Autodesk Fusion 360 part; units mm, degrees
note: some values were not read from the file. Set by a fixed rule: which sketch regions a step uses.
(part 2 of 2)
sketch "Sketch14" plane through (0, 0, 1.5) normal (0, 0, 1) x (-1, 0, 0)
  line L0 (-6.1342, -0.2087) -> (-6.1342, -10.2087)
  line L1 (-6.1342, -10.2087) -> (-9.8859, -10.2087)
  spline S0 degree 3 poles (-9.8859, -10.2087) (-10.2332, -10.2024) (-10.8611, -10.1909) (-11.4553, -9.9911) (-11.7208, -9.9018) knots 0 0 0 0 0.103457 0.187012 0.187012 0.187012 0.187012
  spline S1 degree 3 poles (-11.7208, -9.9018) (-11.9396, -9.7883) (-12.3751, -9.5625) (-12.6625, -9.165) (-12.8054, -8.9673) knots 0 0 0 0 0.07283 0.144951 0.144951 0.144951 0.144951
  spline S2 degree 3 poles (-12.8054, -8.9673) (-12.9208, -8.7579) (-13.1471, -8.3471) (-13.1833, -7.8798) (-13.201, -7.6508) knots 0 0 0 0 0.070808 0.13889 0.13889 0.13889 0.13889
  spline S3 degree 3 poles (-13.201, -7.6508) (-13.186, -7.4393) (-13.1557, -7.0123) (-12.9546, -6.6342) (-12.8532, -6.4434) knots 0 0 0 0 0.062849 0.126897 0.126897 0.126897 0.126897
  spline S4 degree 3 poles (-12.8532, -6.4434) (-12.7177, -6.2615) (-12.4343, -5.881) (-12.0193, -5.6499) (-11.8027, -5.5293) knots 0 0 0 0 0.067255 0.140662 0.140662 0.140662 0.140662
  spline S5 degree 3 poles (-11.8027, -5.5293) (-12.0835, -5.4301) (-12.6217, -5.2399) (-13.009, -4.8219) (-13.1942, -4.6221) knots 0 0 0 0 0.087856 0.168343 0.168343 0.168343 0.168343
  spline S6 degree 3 poles (-13.1942, -4.6221) (-13.3375, -4.3958) (-13.6301, -3.9333) (-13.6667, -3.3868) (-13.6854, -3.1078) knots 0 0 0 0 0.079028 0.161462 0.161462 0.161462 0.161462
  spline S7 degree 3 poles (-13.6854, -3.1078) (-13.6733, -2.8786) (-13.6495, -2.4244) (-13.4728, -2.0055) (-13.3852, -1.7981) knots 0 0 0 0 0.068285 0.135277 0.135277 0.135277 0.135277
  spline S8 degree 3 poles (-13.3852, -1.7981) (-13.2857, -1.6126) (-13.0966, -1.2602) (-12.7972, -0.9957) (-12.6553, -0.8704) knots 0 0 0 0 0.062563 0.118877 0.118877 0.118877 0.118877
  spline S9 degree 3 poles (-12.6553, -0.8704) (-12.4947, -0.7664) (-12.1539, -0.5456) (-11.7635, -0.4324) (-11.5571, -0.3725) knots 0 0 0 0 0.057092 0.121161 0.121161 0.121161 0.121161
  spline S10 degree 3 poles (-11.5571, -0.3725) (-11.3145, -0.3248) (-10.7833, -0.2204) (-10.2416, -0.2129) (-9.9473, -0.2087) knots 0 0 0 0 0.074013 0.162103 0.162103 0.162103 0.162103
  line L2 (-9.9473, -0.2087) -> (-6.1342, -0.2087)
  line L3 (-22.6281, -2.3711) -> (-23.8423, -2.5621)
  spline S11 degree 3 poles (-23.8423, -2.5621) (-23.8868, -2.337) (-23.9714, -1.9101) (-24.2681, -1.5932) (-24.4084, -1.4434) knots 0 0 0 0 0.06728 0.127631 0.127631 0.127631 0.127631
  spline S12 degree 3 poles (-24.4084, -1.4434) (-24.591, -1.3302) (-24.9905, -1.0825) (-25.4621, -1.0644) (-25.7181, -1.0546) knots 0 0 0 0 0.063382 0.138705 0.138705 0.138705 0.138705
  spline S13 degree 3 poles (-25.7181, -1.0546) (-25.9704, -1.0603) (-26.4193, -1.0704) (-26.8045, -1.2966) (-26.9732, -1.3957) knots 0 0 0 0 0.074162 0.131971 0.131971 0.131971 0.131971
  spline S14 degree 3 poles (-26.9732, -1.3957) (-27.0925, -1.5129) (-27.3215, -1.738) (-27.3627, -2.0554) (-27.3825, -2.2074) knots 0 0 0 0 0.048606 0.09328 0.09328 0.09328 0.09328
  spline S15 degree 3 poles (-27.3825, -2.2074) (-27.3667, -2.3392) (-27.3348, -2.606) (-27.1264, -2.7761) (-27.021, -2.8622) knots 0 0 0 0 0.038259 0.077458 0.077458 0.077458 0.077458
  spline S16 degree 3 poles (-27.021, -2.8622) (-26.8755, -2.9276) (-26.472, -3.1087) (-26.0413, -3.2122) (-25.7659, -3.2783) knots 0 0 0 0 0.047763 0.132466 0.132466 0.132466 0.132466
  spline S17 degree 3 poles (-25.7659, -3.2783) (-25.3814, -3.3747) (-24.7446, -3.5343) (-24.1326, -3.7711) (-23.89, -3.865) knots 0 0 0 0 0.118742 0.196704 0.196704 0.196704 0.196704
  spline S18 degree 3 poles (-23.89, -3.865) (-23.7289, -3.9545) (-23.4161, -4.1282) (-23.2024, -4.4149) (-23.0987, -4.5539) knots 0 0 0 0 0.054583 0.105986 0.105986 0.105986 0.105986
  spline S19 degree 3 poles (-23.0987, -4.5539) (-23.0211, -4.7061) (-22.8648, -5.0127) (-22.8434, -5.3563) (-22.8327, -5.5293) knots 0 0 0 0 0.050651 0.102072 0.102072 0.102072 0.102072
  spline S20 degree 3 poles (-22.8327, -5.5293) (-22.8414, -5.6869) (-22.8585, -5.9984) (-22.9873, -6.2825) (-23.051, -6.4229) knots 0 0 0 0 0.046874 0.092701 0.092701 0.092701 0.092701
  spline S21 degree 3 poles (-23.051, -6.4229) (-23.1324, -6.5556) (-23.295, -6.8203) (-23.5372, -7.0148) (-23.6581, -7.1119) knots 0 0 0 0 0.046313 0.092439 0.092439 0.092439 0.092439
  spline S22 degree 3 poles (-23.6581, -7.1119) (-23.7685, -7.1813) (-24.0116, -7.3342) (-24.2859, -7.4198) (-24.4357, -7.4666) knots 0 0 0 0 0.038962 0.085789 0.085789 0.085789 0.085789
  spline S23 degree 3 poles (-24.4357, -7.4666) (-24.6065, -7.5104) (-24.9556, -7.5998) (-25.3158, -7.611) (-25.4998, -7.6167) knots 0 0 0 0 0.052716 0.107755 0.107755 0.107755 0.107755
  spline S24 degree 3 poles (-25.4998, -7.6167) (-25.7686, -7.6089) (-26.2779, -7.5942) (-26.7641, -7.4427) (-26.9937, -7.3711) knots 0 0 0 0 0.080215 0.152023 0.152023 0.152023 0.152023
  spline S25 degree 3 poles (-26.9937, -7.3711) (-27.1909, -7.2879) (-27.5579, -7.133) (-27.825, -6.8387) (-27.9487, -6.7026) knots 0 0 0 0 0.063304 0.117817 0.117817 0.117817 0.117817
  spline S26 degree 3 poles (-27.9487, -6.7026) (-28.0443, -6.5436) (-28.2527, -6.197) (-28.3298, -5.7992) (-28.3716, -5.5839) knots 0 0 0 0 0.055232 0.120418 0.120418 0.120418 0.120418
  line L4 (-28.3716, -5.5839) -> (-27.171, -5.4202)
  spline S27 degree 3 poles (-27.171, -5.4202) (-27.1329, -5.5947) (-27.0588, -5.9329) (-26.8127, -6.1757) (-26.6935, -6.2933) knots 0 0 0 0 0.052312 0.101441 0.101441 0.101441 0.101441
  spline S28 degree 3 poles (-26.6935, -6.2933) (-26.5405, -6.3846) (-26.2017, -6.5868) (-25.8057, -6.5999) (-25.5885, -6.6071) knots 0 0 0 0 0.052622 0.116544 0.116544 0.116544 0.116544
  spline S29 degree 3 poles (-25.5885, -6.6071) (-25.3414, -6.6051) (-24.9157, -6.6017) (-24.5391, -6.4085) (-24.3811, -6.3274) knots 0 0 0 0 0.072813 0.125434 0.125434 0.125434 0.125434
  spline S30 degree 3 poles (-24.3811, -6.3274) (-24.2758, -6.2342) (-24.0766, -6.058) (-24.0379, -5.796) (-24.0196, -5.6726) knots 0 0 0 0 0.040701 0.076975 0.076975 0.076975 0.076975
  spline S31 degree 3 poles (-24.0196, -5.6726) (-24.026, -5.5949) (-24.0388, -5.4386) (-24.1259, -5.3083) (-24.1697, -5.2429) knots 0 0 0 0 0.022989 0.046194 0.046194 0.046194 0.046194
  spline S32 degree 3 poles (-24.1697, -5.2429) (-24.2308, -5.1782) (-24.3646, -5.0367) (-24.5433, -4.9581) (-24.6403, -4.9154) knots 0 0 0 0 0.026422 0.05785 0.05785 0.05785 0.05785
  spline S33 degree 3 poles (-24.6403, -4.9154) (-24.7612, -4.8773) (-25.1203, -4.7642) (-25.4838, -4.6665) (-25.7249, -4.6017) knots 0 0 0 0 0.038027 0.112916 0.112916 0.112916 0.112916
  spline S34 degree 3 poles (-25.7249, -4.6017) (-26.0956, -4.5032) (-26.7095, -4.3403) (-27.3039, -4.1171) (-27.5394, -4.0287) knots 0 0 0 0 0.114967 0.190379 0.190379 0.190379 0.190379
  spline S35 degree 3 poles (-27.5394, -4.0287) (-27.7016, -3.9491) (-28.0185, -3.7937) (-28.242, -3.5207) (-28.3511, -3.3875) knots 0 0 0 0 0.053495 0.104527 0.104527 0.104527 0.104527
  spline S36 degree 3 poles (-28.3511, -3.3875) (-28.4366, -3.2329) (-28.6171, -2.9066) (-28.635, -2.5334) (-28.6444, -2.337) knots 0 0 0 0 0.052263 0.110368 0.110368 0.110368 0.110368
  spline S37 degree 3 poles (-28.6444, -2.337) (-28.6284, -2.1337) (-28.5957, -1.72) (-28.3883, -1.3603) (-28.2829, -1.1774) knots 0 0 0 0 0.060367 0.122834 0.122834 0.122834 0.122834
  spline S38 degree 3 poles (-28.2829, -1.1774) (-28.1475, -1.006) (-27.8666, -0.6506) (-27.4623, -0.4449) (-27.2529, -0.3384) knots 0 0 0 0 0.064709 0.134257 0.134257 0.134257 0.134257
  spline S39 degree 3 poles (-27.2529, -0.3384) (-27.0154, -0.2528) (-26.5218, -0.0751) (-25.9971, -0.0553) (-25.7249, -0.045) knots 0 0 0 0 0.075252 0.156416 0.156416 0.156416 0.156416
  spline S40 degree 3 poles (-25.7249, -0.045) (-25.2992, -0.0571) (-24.5301, -0.079) (-23.866, -0.4611) (-23.5694, -0.6317) knots 0 0 0 0 0.125349 0.226485 0.226485 0.226485 0.226485
  spline S41 degree 3 poles (-23.5694, -0.6317) (-23.3443, -0.8611) (-22.8656, -1.3493) (-22.7103, -2.0172) (-22.6281, -2.3711) knots 0 0 0 0 0.094587 0.201201 0.201201 0.201201 0.201201
  line L5 (-51.0387, -0.2087) -> (-51.0387, -10.2087)
  line L6 (-51.0387, -10.2087) -> (-52.2665, -10.2087)
  line L7 (-52.2665, -10.2087) -> (-52.2665, -0.2087)
  line L8 (-52.2665, -0.2087) -> (-51.0387, -0.2087)
  line L9 (-33.2147, -0.2087) -> (-33.2147, -7.4529)
  line L10 (-33.2147, -7.4529) -> (-34.4425, -7.4529)
  line L11 (-34.4425, -7.4529) -> (-34.4425, -0.2087)
  line L12 (-34.4425, -0.2087) -> (-33.2147, -0.2087)
  spline S42 degree 3 poles (-20.0769, -1.1023) (-19.8601, -0.9267) (-19.4552, -0.5985) (-18.9808, -0.3836) (-18.7604, -0.2838) knots 0 0 0 0 0.08329 0.155589 0.155589 0.155589 0.155589
  spline S43 degree 3 poles (-18.7604, -0.2838) (-18.545, -0.2142) (-18.106, -0.0722) (-17.6448, -0.0542) (-17.4098, -0.045) knots 0 0 0 0 0.067559 0.137732 0.137732 0.137732 0.137732
  spline S44 degree 3 poles (-17.4098, -0.045) (-17.0466, -0.0594) (-16.3791, -0.0858) (-15.8267, -0.4561) (-15.5749, -0.6248) knots 0 0 0 0 0.10655 0.195795 0.195795 0.195795 0.195795
  spline S45 degree 3 poles (-15.5749, -0.6248) (-15.3878, -0.8356) (-15.0092, -1.2622) (-14.959, -1.8309) (-14.9337, -2.1187) knots 0 0 0 0 0.082211 0.166458 0.166458 0.166458 0.166458
  spline S46 degree 3 poles (-14.9337, -2.1187) (-14.9429, -2.2908) (-14.961, -2.6289) (-15.1028, -2.9363) (-15.1724, -3.0873) knots 0 0 0 0 0.051168 0.100571 0.100571 0.100571 0.100571
  spline S47 degree 3 poles (-15.1724, -3.0873) (-15.2589, -3.2269) (-15.4288, -3.5007) (-15.6824, -3.6993) (-15.8068, -3.7967) knots 0 0 0 0 0.048827 0.095831 0.095831 0.095831 0.095831
  spline S48 degree 3 poles (-15.8068, -3.7967) (-15.944, -3.8804) (-16.2232, -4.0506) (-16.535, -4.1491) (-16.6935, -4.1992) knots 0 0 0 0 0.048018 0.0977 0.0977 0.0977 0.0977
  spline S49 degree 3 poles (-16.6935, -4.1992) (-16.8444, -4.2325) (-17.205, -4.312) (-17.5717, -4.3571) (-17.785, -4.3834) knots 0 0 0 0 0.046321 0.110737 0.110737 0.110737 0.110737
  spline S50 degree 3 poles (-17.785, -4.3834) (-18.2178, -4.4358) (-18.958, -4.5254) (-19.6763, -4.7239) (-19.9746, -4.8063) knots 0 0 0 0 0.130548 0.223278 0.223278 0.223278 0.223278
  spline S51 degree 3 poles (-19.9746, -4.8063) (-19.9765, -4.8751) (-19.9795, -4.9819) (-19.9809, -5.0888) (-19.9814, -5.1269) knots 0 0 0 0 0.020641 0.032068 0.032068 0.032068 0.032068
  spline S52 degree 3 poles (-19.9814, -5.1269) (-19.9765, -5.3488) (-19.9679, -5.74) (-19.7345, -6.05) (-19.6335, -6.1842) knots 0 0 0 0 0.064538 0.113796 0.113796 0.113796 0.113796
  spline S53 degree 3 poles (-19.6335, -6.1842) (-19.444, -6.3052) (-19.0199, -6.5759) (-18.5146, -6.5916) (-18.2352, -6.6003) knots 0 0 0 0 0.066297 0.148303 0.148303 0.148303 0.148303
  spline S54 degree 3 poles (-18.2352, -6.6003) (-17.9783, -6.5961) (-17.526, -6.5887) (-17.1257, -6.3824) (-16.9528, -6.2933) knots 0 0 0 0 0.075765 0.133425 0.133425 0.133425 0.133425
  spline S55 degree 3 poles (-16.9528, -6.2933) (-16.8223, -6.161) (-16.5255, -5.8602) (-16.4102, -5.4514) (-16.3457, -5.2224) knots 0 0 0 0 0.054917 0.124877 0.124877 0.124877 0.124877
  line L13 (-16.3457, -5.2224) -> (-15.1451, -5.3861)
  spline S56 degree 3 poles (-15.1451, -5.3861) (-15.2036, -5.6241) (-15.3129, -6.0691) (-15.5662, -6.4503) (-15.684, -6.6276) knots 0 0 0 0 0.07287 0.136248 0.136248 0.136248 0.136248
  spline S57 degree 3 poles (-15.684, -6.6276) (-15.8291, -6.7794) (-16.1367, -7.1015) (-16.5501, -7.2689) (-16.7686, -7.3575) knots 0 0 0 0 0.062278 0.132061 0.132061 0.132061 0.132061
  spline S58 degree 3 poles (-16.7686, -7.3575) (-17.0221, -7.433) (-17.5581, -7.5927) (-18.1176, -7.6084) (-18.4125, -7.6167) knots 0 0 0 0 0.078998 0.167061 0.167061 0.167061 0.167061
  spline S59 degree 3 poles (-18.4125, -7.6167) (-18.6948, -7.6119) (-19.2072, -7.6033) (-19.6991, -7.4619) (-19.92, -7.3984) knots 0 0 0 0 0.084249 0.152908 0.152908 0.152908 0.152908
  spline S60 degree 3 poles (-19.92, -7.3984) (-20.0951, -7.327) (-20.4151, -7.1966) (-20.6612, -6.9552) (-20.7727, -6.8459) knots 0 0 0 0 0.056055 0.102466 0.102466 0.102466 0.102466
  spline S61 degree 3 poles (-20.7727, -6.8459) (-20.8576, -6.7255) (-21.0364, -6.4721) (-21.1139, -6.1715) (-21.1547, -6.0137) knots 0 0 0 0 0.043817 0.092245 0.092245 0.092245 0.092245
  spline S62 degree 3 poles (-21.1547, -6.0137) (-21.1724, -5.8672) (-21.2178, -5.4913) (-21.2167, -5.1125) (-21.2161, -4.8813) knots 0 0 0 0 0.044238 0.113491 0.113491 0.113491 0.113491
  line L14 (-21.2161, -4.8813) -> (-21.2161, -3.2442)
  spline S63 degree 3 poles (-21.2161, -3.2442) (-21.2134, -2.7777) (-21.2093, -2.0534) (-21.2696, -1.3319) (-21.2911, -1.075) knots 0 0 0 0 0.139849 0.217135 0.217135 0.217135 0.217135
  spline S64 degree 3 poles (-21.2911, -1.075) (-21.325, -0.9257) (-21.3936, -0.6239) (-21.534, -0.3481) (-21.6049, -0.2087) knots 0 0 0 0 0.045752 0.092454 0.092454 0.092454 0.092454
  line L15 (-21.6049, -0.2087) -> (-20.3225, -0.2087)
  spline S65 degree 3 poles (-20.3225, -0.2087) (-20.2641, -0.3452) (-20.1416, -0.6317) (-20.0991, -0.9406) (-20.0769, -1.1023) knots 0 0 0 0 0.04431 0.093043 0.093043 0.093043 0.093043
  arc A0 (15.7488, -13.8378) -> (20.7488, -8.8378) centre (15.7488, -8.8378) ccw
  line L16 (20.7488, -8.8378) -> (20.7488, 93.1622)
  arc A1 (20.7488, 93.1622) -> (15.7488, 98.1622) centre (15.7488, 93.1622) ccw
  line L17 (15.7488, 98.1622) -> (-73.2512, 98.1622)
  arc A2 (-73.2512, 98.1622) -> (-78.2512, 93.1622) centre (-73.2512, 93.1622) ccw
  line L18 (-78.2512, 93.1622) -> (-78.2512, -8.8378)
  arc A3 (-78.2512, -8.8378) -> (-73.2512, -13.8378) centre (-73.2512, -8.8378) ccw
  line L19 (-73.2512, -13.8378) -> (15.7488, -13.8378)
  circle A4 centre (-73.2512, -8.8378) radius 1.7
  circle A5 centre (15.7488, 93.1622) radius 1.7
  line L20 (-3.6362, 61.1472) -> (-16.6362, 61.1472)
  arc A6 (-17.1362, 61.6472) -> (-16.6362, 61.1472) centre (-16.6362, 61.6472) ccw
  line L21 (-17.1362, 61.6472) -> (-17.1362, 74.6472)
  arc A7 (-16.6362, 75.1472) -> (-17.1362, 74.6472) centre (-16.6362, 74.6472) ccw
  line L22 (-16.6362, 75.1472) -> (-3.6362, 75.1472)
  arc A8 (-3.1362, 74.6472) -> (-3.6362, 75.1472) centre (-3.6362, 74.6472) ccw
  line L23 (-3.1362, 74.6472) -> (-3.1362, 61.6472)
  arc A9 (-3.6362, 61.1472) -> (-3.1362, 61.6472) centre (-3.6362, 61.6472) ccw
  line L24 (-22.6862, 42.0972) -> (-35.6862, 42.0972)
  arc A10 (-36.1862, 42.5972) -> (-35.6862, 42.0972) centre (-35.6862, 42.5972) ccw
  line L25 (-36.1862, 42.5972) -> (-36.1862, 55.5972)
  arc A11 (-35.6862, 56.0972) -> (-36.1862, 55.5972) centre (-35.6862, 55.5972) ccw
  line L26 (-35.6862, 56.0972) -> (-22.6862, 56.0972)
  arc A12 (-22.1862, 55.5972) -> (-22.6862, 56.0972) centre (-22.6862, 55.5972) ccw
  line L27 (-22.1862, 55.5972) -> (-22.1862, 42.5972)
  arc A13 (-22.6862, 42.0972) -> (-22.1862, 42.5972) centre (-22.6862, 42.5972) ccw
  line L28 (-41.7362, 23.0472) -> (-54.7362, 23.0472)
  arc A14 (-55.2362, 23.5472) -> (-54.7362, 23.0472) centre (-54.7362, 23.5472) ccw
  line L29 (-55.2362, 23.5472) -> (-55.2362, 36.5472)
  arc A15 (-54.7362, 37.0472) -> (-55.2362, 36.5472) centre (-54.7362, 36.5472) ccw
  line L30 (-54.7362, 37.0472) -> (-41.7362, 37.0472)
  arc A16 (-41.2362, 36.5472) -> (-41.7362, 37.0472) centre (-41.7362, 36.5472) ccw
  line L31 (-41.2362, 36.5472) -> (-41.2362, 23.5472)
  arc A17 (-41.7362, 23.0472) -> (-41.2362, 23.5472) centre (-41.7362, 23.5472) ccw
  line L32 (-3.6362, 42.0972) -> (-16.6362, 42.0972)
  arc A18 (-17.1362, 42.5972) -> (-16.6362, 42.0972) centre (-16.6362, 42.5972) ccw
  line L33 (-17.1362, 42.5972) -> (-17.1362, 55.5972)
  arc A19 (-16.6362, 56.0972) -> (-17.1362, 55.5972) centre (-16.6362, 55.5972) ccw
  line L34 (-16.6362, 56.0972) -> (-3.6362, 56.0972)
  arc A20 (-3.1362, 55.5972) -> (-3.6362, 56.0972) centre (-3.6362, 55.5972) ccw
  line L35 (-3.1362, 55.5972) -> (-3.1362, 42.5972)
  arc A21 (-3.6362, 42.0972) -> (-3.1362, 42.5972) centre (-3.6362, 42.5972) ccw
  line L36 (-22.6862, 61.1472) -> (-35.6862, 61.1472)
  arc A22 (-36.1862, 61.6472) -> (-35.6862, 61.1472) centre (-35.6862, 61.6472) ccw
  line L37 (-36.1862, 61.6472) -> (-36.1862, 74.6472)
  arc A23 (-35.6862, 75.1472) -> (-36.1862, 74.6472) centre (-35.6862, 74.6472) ccw
  line L38 (-35.6862, 75.1472) -> (-22.6862, 75.1472)
  arc A24 (-22.1862, 74.6472) -> (-22.6862, 75.1472) centre (-22.6862, 74.6472) ccw
  line L39 (-22.1862, 74.6472) -> (-22.1862, 61.6472)
  arc A25 (-22.6862, 61.1472) -> (-22.1862, 61.6472) centre (-22.6862, 61.6472) ccw
  line L40 (-41.7362, 42.0972) -> (-54.7362, 42.0972)
  arc A26 (-55.2362, 42.5972) -> (-54.7362, 42.0972) centre (-54.7362, 42.5972) ccw
  line L41 (-55.2362, 42.5972) -> (-55.2362, 55.5972)
  arc A27 (-54.7362, 56.0972) -> (-55.2362, 55.5972) centre (-54.7362, 55.5972) ccw
  line L42 (-54.7362, 56.0972) -> (-41.7362, 56.0972)
  arc A28 (-41.2362, 55.5972) -> (-41.7362, 56.0972) centre (-41.7362, 55.5972) ccw
  line L43 (-41.2362, 55.5972) -> (-41.2362, 42.5972)
  arc A29 (-41.7362, 42.0972) -> (-41.2362, 42.5972) centre (-41.7362, 42.5972) ccw
  line L44 (-22.6862, 23.0472) -> (-35.6862, 23.0472)
  arc A30 (-36.1862, 23.5472) -> (-35.6862, 23.0472) centre (-35.6862, 23.5472) ccw
  line L45 (-36.1862, 23.5472) -> (-36.1862, 36.5472)
  arc A31 (-35.6862, 37.0472) -> (-36.1862, 36.5472) centre (-35.6862, 36.5472) ccw
  line L46 (-35.6862, 37.0472) -> (-22.6862, 37.0472)
  arc A32 (-22.1862, 36.5472) -> (-22.6862, 37.0472) centre (-22.6862, 36.5472) ccw
  line L47 (-22.1862, 36.5472) -> (-22.1862, 23.5472)
  arc A33 (-22.6862, 23.0472) -> (-22.1862, 23.5472) centre (-22.6862, 23.5472) ccw
  line L48 (-3.6362, 23.0472) -> (-16.6362, 23.0472)
  arc A34 (-17.1362, 23.5472) -> (-16.6362, 23.0472) centre (-16.6362, 23.5472) ccw
  line L49 (-17.1362, 23.5472) -> (-17.1362, 36.5472)
  arc A35 (-16.6362, 37.0472) -> (-17.1362, 36.5472) centre (-16.6362, 36.5472) ccw
  line L50 (-16.6362, 37.0472) -> (-3.6362, 37.0472)
  arc A36 (-3.1362, 36.5472) -> (-3.6362, 37.0472) centre (-3.6362, 36.5472) ccw
  line L51 (-3.1362, 36.5472) -> (-3.1362, 23.5472)
  arc A37 (-3.6362, 23.0472) -> (-3.1362, 23.5472) centre (-3.6362, 23.5472) ccw
  line L52 (-41.7362, 61.1472) -> (-54.7362, 61.1472)
  arc A38 (-55.2362, 61.6472) -> (-54.7362, 61.1472) centre (-54.7362, 61.6472) ccw
  line L53 (-55.2362, 61.6472) -> (-55.2362, 74.6472)
  arc A39 (-54.7362, 75.1472) -> (-55.2362, 74.6472) centre (-54.7362, 74.6472) ccw
  line L54 (-54.7362, 75.1472) -> (-41.7362, 75.1472)
  arc A40 (-41.2362, 74.6472) -> (-41.7362, 75.1472) centre (-41.7362, 74.6472) ccw
  line L55 (-41.2362, 74.6472) -> (-41.2362, 61.6472)
  arc A41 (-41.7362, 61.1472) -> (-41.2362, 61.6472) centre (-41.7362, 61.6472) ccw
  circle A42 centre (15.7488, -8.8378) radius 1.7
  circle A43 centre (-73.2512, 93.1622) radius 1.7
  circle A44 centre (-10.3772, 7.104) radius 4.5
  circle A45 centre (-48.3914, 7.0872) radius 4.75
  line L56 (-19.9185, 7.8179) -> (-19.2596, 9.6351)
  line L57 (-19.2596, 9.6351) -> (-18.4165, 9.6351)
  line L58 (-18.4165, 9.6351) -> (-20.7207, 3.6351)
  line L59 (-20.7207, 3.6351) -> (-21.5761, 3.6351)
  line L60 (-21.5761, 3.6351) -> (-24.0317, 9.6351)
  line L61 (-24.0317, 9.6351) -> (-23.1272, 9.6351)
  line L62 (-23.1272, 9.6351) -> (-22.4274, 7.8179)
  line L63 (-22.4274, 7.8179) -> (-19.9185, 7.8179)
  line L64 (-36.9526, 7.2572) -> (-36.9526, 9.6351)
  line L65 (-36.9526, 9.6351) -> (-36.2159, 9.6351)
  line L66 (-36.2159, 9.6351) -> (-36.2159, 3.6351)
  line L67 (-36.2159, 3.6351) -> (-36.9526, 3.6351)
  line L68 (-36.9526, 3.6351) -> (-36.9526, 5.7879)
  spline S66 degree 3 poles (-36.9526, 5.7879) (-37.1356, 5.6137) (-37.5011, 5.2655) (-38.0033, 5.2154) (-38.2541, 5.1904) knots 0 0 0 0 0.073552 0.146917 0.146917 0.146917 0.146917
  spline S67 degree 3 poles (-38.2541, 5.1904) (-38.4068, 5.1968) (-38.6987, 5.2091) (-38.9657, 5.3267) (-39.0931, 5.3827) knots 0 0 0 0 0.045378 0.086754 0.086754 0.086754 0.086754
  spline S68 degree 3 poles (-39.0931, 5.3827) (-39.2026, 5.4502) (-39.4164, 5.582) (-39.5402, 5.8002) (-39.6006, 5.9066) knots 0 0 0 0 0.0379 0.073998 0.073998 0.073998 0.073998
  spline S69 degree 3 poles (-39.6006, 5.9066) (-39.6458, 6.0426) (-39.7505, 6.3581) (-39.7541, 6.6912) (-39.7562, 6.8807) knots 0 0 0 0 0.042754 0.099164 0.099164 0.099164 0.099164
  line L69 (-39.7562, 6.8807) -> (-39.7562, 9.6351)
  line L70 (-39.7562, 9.6351) -> (-39.0195, 9.6351)
  line L71 (-39.0195, 9.6351) -> (-39.0195, 6.8807)
  spline S70 degree 3 poles (-39.0195, 6.8807) (-39.0156, 6.7164) (-39.0088, 6.4249) (-38.8481, 6.1838) (-38.778, 6.0785) knots 0 0 0 0 0.048061 0.085299 0.085299 0.085299 0.085299
  spline S71 degree 3 poles (-38.778, 6.0785) (-38.6863, 6.0046) (-38.49, 5.8464) (-38.2373, 5.8323) (-38.1027, 5.8248) knots 0 0 0 0 0.03448 0.073774 0.073774 0.073774 0.073774
  spline S72 degree 3 poles (-38.1027, 5.8248) (-37.9947, 5.8322) (-37.7769, 5.8471) (-37.5826, 5.9465) (-37.4847, 5.9967) knots 0 0 0 0 0.03211 0.064744 0.064744 0.064744 0.064744
  spline S73 degree 3 poles (-37.4847, 5.9967) (-37.3963, 6.057) (-37.2219, 6.1761) (-37.1238, 6.3629) (-37.0754, 6.4551) knots 0 0 0 0 0.031576 0.062292 0.062292 0.062292 0.062292
  spline S74 degree 3 poles (-37.0754, 6.4551) (-37.0397, 6.5695) (-36.9585, 6.8302) (-36.9547, 7.1038) (-36.9526, 7.2572) knots 0 0 0 0 0.035789 0.081526 0.081526 0.081526 0.081526
  spline S75 degree 3 poles (-33.5884, 9.7334) (-33.3329, 9.7261) (-32.8715, 9.713) (-32.473, 9.4837) (-32.295, 9.3814) knots 0 0 0 0 0.07521 0.135891 0.135891 0.135891 0.135891
  spline S76 degree 3 poles (-32.295, 9.3814) (-32.16, 9.2437) (-31.8728, 8.9508) (-31.7796, 8.5501) (-31.7302, 8.3377) knots 0 0 0 0 0.056752 0.12072 0.12072 0.12072 0.12072
  line L72 (-31.7302, 8.3377) -> (-32.4588, 8.2231)
  spline S77 degree 3 poles (-32.4588, 8.2231) (-32.4855, 8.3582) (-32.5362, 8.6144) (-32.7143, 8.8045) (-32.7985, 8.8943) knots 0 0 0 0 0.040368 0.076579 0.076579 0.076579 0.076579
  spline S78 degree 3 poles (-32.7985, 8.8943) (-32.908, 8.9623) (-33.1477, 9.1109) (-33.4306, 9.1217) (-33.5843, 9.1276) knots 0 0 0 0 0.038029 0.083223 0.083223 0.083223 0.083223
  spline S79 degree 3 poles (-33.5843, 9.1276) (-33.7356, 9.1242) (-34.005, 9.1182) (-34.2361, 8.9824) (-34.3373, 8.923) knots 0 0 0 0 0.044497 0.079182 0.079182 0.079182 0.079182
  spline S80 degree 3 poles (-34.3373, 8.923) (-34.4089, 8.8526) (-34.5463, 8.7176) (-34.571, 8.5272) (-34.5829, 8.436) knots 0 0 0 0 0.029164 0.055968 0.055968 0.055968 0.055968
  spline S81 degree 3 poles (-34.5829, 8.436) (-34.5734, 8.3569) (-34.5543, 8.1968) (-34.4292, 8.0947) (-34.366, 8.0431) knots 0 0 0 0 0.022955 0.046475 0.046475 0.046475 0.046475
  spline S82 degree 3 poles (-34.366, 8.0431) (-34.2787, 8.0039) (-34.0366, 7.8951) (-33.7782, 7.8331) (-33.6129, 7.7934) knots 0 0 0 0 0.028658 0.079479 0.079479 0.079479 0.079479
  spline S83 degree 3 poles (-33.6129, 7.7934) (-33.3822, 7.7356) (-33.0001, 7.6398) (-32.6329, 7.4977) (-32.4874, 7.4414) knots 0 0 0 0 0.071245 0.118022 0.118022 0.118022 0.118022
  spline S84 degree 3 poles (-32.4874, 7.4414) (-32.3907, 7.3877) (-32.203, 7.2834) (-32.0748, 7.1115) (-32.0126, 7.028) knots 0 0 0 0 0.03275 0.063592 0.063592 0.063592 0.063592
  spline S85 degree 3 poles (-32.0126, 7.028) (-31.9661, 6.9368) (-31.8723, 6.7528) (-31.8595, 6.5466) (-31.853, 6.4428) knots 0 0 0 0 0.03039 0.061243 0.061243 0.061243 0.061243
  spline S86 degree 3 poles (-31.853, 6.4428) (-31.8582, 6.3483) (-31.8685, 6.1613) (-31.9458, 5.9909) (-31.984, 5.9066) knots 0 0 0 0 0.028124 0.055621 0.055621 0.055621 0.055621
  spline S87 degree 3 poles (-31.984, 5.9066) (-32.0329, 5.827) (-32.1304, 5.6682) (-32.2757, 5.5515) (-32.3482, 5.4933) knots 0 0 0 0 0.027788 0.055463 0.055463 0.055463 0.055463
  spline S88 degree 3 poles (-32.3482, 5.4933) (-32.4145, 5.4516) (-32.5603, 5.3599) (-32.725, 5.3085) (-32.8148, 5.2804) knots 0 0 0 0 0.023377 0.051473 0.051473 0.051473 0.051473
  spline S89 degree 3 poles (-32.8148, 5.2804) (-32.9173, 5.2542) (-33.1267, 5.2005) (-33.3429, 5.1938) (-33.4533, 5.1904) knots 0 0 0 0 0.03163 0.064653 0.064653 0.064653 0.064653
  spline S90 degree 3 poles (-33.4533, 5.1904) (-33.6145, 5.1951) (-33.9201, 5.2039) (-34.2118, 5.2948) (-34.3496, 5.3377) knots 0 0 0 0 0.048129 0.091214 0.091214 0.091214 0.091214
  spline S91 degree 3 poles (-34.3496, 5.3377) (-34.4679, 5.3877) (-34.6881, 5.4806) (-34.8484, 5.6571) (-34.9226, 5.7388) knots 0 0 0 0 0.037982 0.07069 0.07069 0.07069 0.07069
  spline S92 degree 3 poles (-34.9226, 5.7388) (-34.98, 5.8342) (-35.105, 6.0422) (-35.1513, 6.2808) (-35.1764, 6.41) knots 0 0 0 0 0.033139 0.072251 0.072251 0.072251 0.072251
  line L73 (-35.1764, 6.41) -> (-34.456, 6.5083)
  spline S93 degree 3 poles (-34.456, 6.5083) (-34.4331, 6.4036) (-34.3887, 6.2006) (-34.241, 6.0549) (-34.1695, 5.9844) knots 0 0 0 0 0.031387 0.060864 0.060864 0.060864 0.060864
  spline S94 degree 3 poles (-34.1695, 5.9844) (-34.0777, 5.9296) (-33.8744, 5.8083) (-33.6368, 5.8004) (-33.5065, 5.7961) knots 0 0 0 0 0.031573 0.069926 0.069926 0.069926 0.069926
  spline S95 degree 3 poles (-33.5065, 5.7961) (-33.3582, 5.7973) (-33.1028, 5.7994) (-32.8769, 5.9153) (-32.7821, 5.9639) knots 0 0 0 0 0.043688 0.075261 0.075261 0.075261 0.075261
  spline S96 degree 3 poles (-32.7821, 5.9639) (-32.7189, 6.0198) (-32.5993, 6.1256) (-32.5761, 6.2828) (-32.5652, 6.3568) knots 0 0 0 0 0.024421 0.046185 0.046185 0.046185 0.046185
  spline S97 degree 3 poles (-32.5652, 6.3568) (-32.569, 6.4035) (-32.5767, 6.4972) (-32.6289, 6.5754) (-32.6552, 6.6147) knots 0 0 0 0 0.013793 0.027717 0.027717 0.027717 0.027717
  spline S98 degree 3 poles (-32.6552, 6.6147) (-32.6919, 6.6535) (-32.7722, 6.7384) (-32.8794, 6.7855) (-32.9376, 6.8111) knots 0 0 0 0 0.015853 0.03471 0.03471 0.03471 0.03471
  spline S99 degree 3 poles (-32.9376, 6.8111) (-33.0102, 6.834) (-33.2256, 6.9019) (-33.4437, 6.9605) (-33.5884, 6.9994) knots 0 0 0 0 0.022816 0.06775 0.06775 0.06775 0.06775
  spline S100 degree 3 poles (-33.5884, 6.9994) (-33.8108, 7.0584) (-34.1791, 7.1562) (-34.5358, 7.2901) (-34.677, 7.3432) knots 0 0 0 0 0.06898 0.114227 0.114227 0.114227 0.114227
  spline S101 degree 3 poles (-34.677, 7.3432) (-34.7744, 7.3909) (-34.9645, 7.4842) (-35.0986, 7.648) (-35.1641, 7.7279) knots 0 0 0 0 0.032097 0.062716 0.062716 0.062716 0.062716
  spline S102 degree 3 poles (-35.1641, 7.7279) (-35.2154, 7.8206) (-35.3237, 8.0164) (-35.3344, 8.2403) (-35.3401, 8.3582) knots 0 0 0 0 0.031358 0.066221 0.066221 0.066221 0.066221
  spline S103 degree 3 poles (-35.3401, 8.3582) (-35.3304, 8.4802) (-35.3108, 8.7284) (-35.1864, 8.9442) (-35.1231, 9.054) knots 0 0 0 0 0.03622 0.0737 0.0737 0.0737 0.0737
  spline S104 degree 3 poles (-35.1231, 9.054) (-35.0419, 9.1568) (-34.8733, 9.37) (-34.6308, 9.4935) (-34.5051, 9.5574) knots 0 0 0 0 0.038826 0.080554 0.080554 0.080554 0.080554
  spline S105 degree 3 poles (-34.5051, 9.5574) (-34.3626, 9.6087) (-34.0665, 9.7153) (-33.7517, 9.7272) (-33.5884, 9.7334) knots 0 0 0 0 0.045151 0.09385 0.09385 0.09385 0.09385
  line L74 (-30.8708, 5.2886) -> (-30.8708, 9.6351)
  line L75 (-30.8708, 9.6351) -> (-30.2118, 9.6351)
  line L76 (-30.2118, 9.6351) -> (-30.2118, 8.9967)
  spline S106 degree 3 poles (-30.2118, 8.9967) (-30.0286, 9.2115) (-29.665, 9.638) (-29.1086, 9.7017) (-28.8326, 9.7334) knots 0 0 0 0 0.08146 0.161672 0.161672 0.161672 0.161672
  spline S107 degree 3 poles (-28.8326, 9.7334) (-28.7071, 9.7275) (-28.4592, 9.716) (-28.2269, 9.629) (-28.1122, 9.586) knots 0 0 0 0 0.037426 0.073927 0.073927 0.073927 0.073927
  spline S108 degree 3 poles (-28.1122, 9.586) (-28.0111, 9.5369) (-27.8224, 9.4452) (-27.6821, 9.2898) (-27.617, 9.2177) knots 0 0 0 0 0.033365 0.062234 0.062234 0.062234 0.062234
  spline S109 degree 3 poles (-27.617, 9.2177) (-27.5673, 9.1363) (-27.463, 8.9656) (-27.4163, 8.771) (-27.3919, 8.6692) knots 0 0 0 0 0.028434 0.059609 0.059609 0.059609 0.059609
  spline S110 degree 3 poles (-27.3919, 8.6692) (-27.3789, 8.5759) (-27.3471, 8.348) (-27.3469, 8.1177) (-27.3469, 7.9817) knots 0 0 0 0 0.028238 0.068977 0.068977 0.068977 0.068977
  line L77 (-27.3469, 7.9817) -> (-27.3469, 5.2886)
  line L78 (-27.3469, 5.2886) -> (-28.0836, 5.2886)
  line L79 (-28.0836, 5.2886) -> (-28.0836, 7.6993)
  spline S111 degree 3 poles (-28.0836, 7.6993) (-28.0828, 7.8606) (-28.0816, 8.1209) (-28.1156, 8.3788) (-28.1286, 8.4769) knots 0 0 0 0 0.048308 0.077969 0.077969 0.077969 0.077969
  spline S112 degree 3 poles (-28.1286, 8.4769) (-28.1576, 8.5681) (-28.2147, 8.7476) (-28.3545, 8.8734) (-28.4233, 8.9353) knots 0 0 0 0 0.028161 0.055379 0.055379 0.055379 0.055379
  spline S113 degree 3 poles (-28.4233, 8.9353) (-28.5051, 8.983) (-28.6769, 9.0831) (-28.8758, 9.0935) (-28.9799, 9.099) knots 0 0 0 0 0.028006 0.05877 0.05877 0.05877 0.05877
  spline S114 degree 3 poles (-28.9799, 9.099) (-29.0889, 9.0919) (-29.3075, 9.0777) (-29.5036, 8.9801) (-29.602, 8.9312) knots 0 0 0 0 0.032401 0.065009 0.065009 0.065009 0.065009
  spline S115 degree 3 poles (-29.602, 8.9312) (-29.6913, 8.8699) (-29.8664, 8.7498) (-29.9636, 8.5612) (-30.0113, 8.4687) knots 0 0 0 0 0.031928 0.062622 0.062622 0.062622 0.062622
  spline S116 degree 3 poles (-30.0113, 8.4687) (-30.0469, 8.3494) (-30.1297, 8.0723) (-30.1325, 7.7825) (-30.1341, 7.6174) knots 0 0 0 0 0.037175 0.086384 0.086384 0.086384 0.086384
  line L80 (-30.1341, 7.6174) -> (-30.1341, 5.2886)
  line L81 (-30.1341, 5.2886) -> (-30.8708, 5.2886)
  line L82 (-25.3005, 7.3596) -> (-25.3005, 9.6351)
  line L83 (-25.3005, 9.6351) -> (-24.5638, 9.6351)
  line L84 (-24.5638, 9.6351) -> (-24.5638, 5.2886)
  line L85 (-24.5638, 5.2886) -> (-25.2268, 5.2886)
  line L86 (-25.2268, 5.2886) -> (-25.2268, 5.9476)
  spline S117 degree 3 poles (-25.2268, 5.9476) (-25.3006, 5.8138) (-25.4259, 5.5864) (-25.6154, 5.4102) (-25.6934, 5.3377) knots 0 0 0 0 0.045445 0.077208 0.077208 0.077208 0.077208
  spline S118 degree 3 poles (-25.6934, 5.3377) (-25.7672, 5.2948) (-25.9142, 5.2092) (-26.0838, 5.1966) (-26.1682, 5.1904) knots 0 0 0 0 0.02526 0.050294 0.050294 0.050294 0.050294
  spline S119 degree 3 poles (-26.1682, 5.1904) (-26.2958, 5.2022) (-26.5648, 5.227) (-26.8011, 5.3586) (-26.9253, 5.4278) knots 0 0 0 0 0.038017 0.080131 0.080131 0.080131 0.080131
  line L87 (-26.9253, 5.4278) -> (-26.6716, 6.1113)
  spline S120 degree 3 poles (-26.6716, 6.1113) (-26.5835, 6.0647) (-26.4139, 5.9752) (-26.223, 5.9593) (-26.1313, 5.9516) knots 0 0 0 0 0.029546 0.056852 0.056852 0.056852 0.056852
  spline S121 degree 3 poles (-26.1313, 5.9516) (-26.0529, 5.9578) (-25.8958, 5.9701) (-25.7636, 6.056) (-25.6975, 6.099) knots 0 0 0 0 0.023214 0.04647 0.04647 0.04647 0.04647
  spline S122 degree 3 poles (-25.6975, 6.099) (-25.6376, 6.1528) (-25.5137, 6.2641) (-25.4541, 6.4197) (-25.4233, 6.5001) knots 0 0 0 0 0.023809 0.049209 0.049209 0.049209 0.049209
  spline S123 degree 3 poles (-25.4233, 6.5001) (-25.3875, 6.6364) (-25.3135, 6.9181) (-25.3049, 7.2093) (-25.3005, 7.3596) knots 0 0 0 0 0.042151 0.087071 0.087071 0.087071 0.087071
  line L88 (-30.0769, -0.2087) -> (-30.0769, -10.2087)
  line L89 (-30.0769, -10.2087) -> (-31.3047, -10.2087)
  line L90 (-31.3047, -10.2087) -> (-31.3047, -0.2087)
  line L91 (-31.3047, -0.2087) -> (-30.0769, -0.2087)
  line L92 (-33.2147, -8.7967) -> (-33.2147, -10.2087)
  line L93 (-33.2147, -10.2087) -> (-34.4425, -10.2087)
  line L94 (-34.4425, -10.2087) -> (-34.4425, -8.7967)
  line L95 (-34.4425, -8.7967) -> (-33.2147, -8.7967)
  line L96 (-36.257, 2.5812) -> (-36.1206, 1.4284)
  spline S124 degree 3 poles (-36.1206, 1.4284) (-36.2455, 1.4601) (-36.4764, 1.5188) (-36.7141, 1.5316) (-36.8231, 1.5375) knots 0 0 0 0 0.038566 0.071252 0.071252 0.071252 0.071252
  spline S125 degree 3 poles (-36.8231, 1.5375) (-36.9478, 1.5344) (-37.1748, 1.5287) (-37.3837, 1.4408) (-37.478, 1.4011) knots 0 0 0 0 0.036992 0.067414 0.067414 0.067414 0.067414
  spline S126 degree 3 poles (-37.478, 1.4011) (-37.5564, 1.3507) (-37.7147, 1.2489) (-37.8249, 1.0962) (-37.8804, 1.0191) knots 0 0 0 0 0.027696 0.055929 0.055929 0.055929 0.055929
  spline S127 degree 3 poles (-37.8804, 1.0191) (-37.9326, 0.9129) (-38.0781, 0.6169) (-38.1863, 0.305) (-38.2556, 0.105) knots 0 0 0 0 0.035471 0.098882 0.098882 0.098882 0.098882
  spline S128 degree 3 poles (-38.2556, 0.105) (-38.2702, 0.0629) (-38.3051, -0.0377) (-38.3428, -0.1372) (-38.3648, -0.1951) knots 0 0 0 0 0.013376 0.031938 0.031938 0.031938 0.031938
  line L97 (-38.3648, -0.1951) -> (-35.6158, -7.4529)
  line L98 (-35.6158, -7.4529) -> (-36.9391, -7.4529)
  line L99 (-36.9391, -7.4529) -> (-38.4466, -3.2579)
  spline S129 degree 3 poles (-38.4466, -3.2579) (-38.5425, -2.986) (-38.7375, -2.4329) (-38.8928, -1.8674) (-38.9719, -1.5798) knots 0 0 0 0 0.086446 0.175881 0.175881 0.175881 0.175881
  spline S130 degree 3 poles (-38.9719, -1.5798) (-39.0455, -1.8595) (-39.1922, -2.4163) (-39.3821, -2.96) (-39.4766, -3.2306) knots 0 0 0 0 0.08672 0.172679 0.172679 0.172679 0.172679
  line L100 (-39.4766, -3.2306) -> (-41.0251, -7.4529)
  line L101 (-41.0251, -7.4529) -> (-42.2529, -7.4529)
  line L102 (-42.2529, -7.4529) -> (-39.4971, -0.086)
  spline S131 degree 3 poles (-39.4971, -0.086) (-39.372, 0.2526) (-39.1658, 0.8106) (-38.9091, 1.347) (-38.8081, 1.558) knots 0 0 0 0 0.10821 0.178327 0.178327 0.178327 0.178327
  spline S132 degree 3 poles (-38.8081, 1.558) (-38.7016, 1.7421) (-38.5042, 2.0832) (-38.1985, 2.3308) (-38.0578, 2.4447) knots 0 0 0 0 0.063189 0.117035 0.117035 0.117035 0.117035
  spline S133 degree 3 poles (-38.0578, 2.4447) (-37.9066, 2.5283) (-37.5927, 2.7017) (-37.2342, 2.7212) (-37.0483, 2.7312) knots 0 0 0 0 0.05112 0.106158 0.106158 0.106158 0.106158
  spline S134 degree 3 poles (-37.0483, 2.7312) (-36.9223, 2.7235) (-36.6524, 2.7068) (-36.3945, 2.6249) (-36.257, 2.5812) knots 0 0 0 0 0.037704 0.080809 0.080809 0.080809 0.080809
  spline S135 degree 3 poles (-48.0237, -1.1023) (-47.8069, -0.9267) (-47.402, -0.5985) (-46.9276, -0.3836) (-46.7072, -0.2838) knots 0 0 0 0 0.08329 0.155589 0.155589 0.155589 0.155589
  spline S136 degree 3 poles (-46.7072, -0.2838) (-46.4918, -0.2142) (-46.0528, -0.0722) (-45.5916, -0.0542) (-45.3566, -0.045) knots 0 0 0 0 0.067559 0.137732 0.137732 0.137732 0.137732
  spline S137 degree 3 poles (-45.3566, -0.045) (-44.9934, -0.0594) (-44.3259, -0.0858) (-43.7735, -0.4561) (-43.5217, -0.6248) knots 0 0 0 0 0.10655 0.195794 0.195794 0.195794 0.195794
  spline S138 degree 3 poles (-43.5217, -0.6248) (-43.3346, -0.8356) (-42.956, -1.2622) (-42.9058, -1.8309) (-42.8804, -2.1187) knots 0 0 0 0 0.082211 0.166458 0.166458 0.166458 0.166458
  spline S139 degree 3 poles (-42.8804, -2.1187) (-42.8897, -2.2908) (-42.9078, -2.6289) (-43.0496, -2.9363) (-43.1192, -3.0873) knots 0 0 0 0 0.051168 0.100571 0.100571 0.100571 0.100571
  spline S140 degree 3 poles (-43.1192, -3.0873) (-43.2057, -3.2269) (-43.3756, -3.5007) (-43.6292, -3.6993) (-43.7536, -3.7967) knots 0 0 0 0 0.048827 0.095831 0.095831 0.095831 0.095831
  spline S141 degree 3 poles (-43.7536, -3.7967) (-43.8908, -3.8804) (-44.17, -4.0506) (-44.4818, -4.1491) (-44.6403, -4.1992) knots 0 0 0 0 0.048018 0.0977 0.0977 0.0977 0.0977
  spline S142 degree 3 poles (-44.6403, -4.1992) (-44.7912, -4.2325) (-45.1518, -4.312) (-45.5185, -4.3571) (-45.7317, -4.3834) knots 0 0 0 0 0.046321 0.110737 0.110737 0.110737 0.110737
  spline S143 degree 3 poles (-45.7317, -4.3834) (-46.1646, -4.4358) (-46.9048, -4.5254) (-47.6231, -4.7239) (-47.9214, -4.8063) knots 0 0 0 0 0.130548 0.223278 0.223278 0.223278 0.223278
  spline S144 degree 3 poles (-47.9214, -4.8063) (-47.9233, -4.8751) (-47.9263, -4.9819) (-47.9277, -5.0888) (-47.9282, -5.1269) knots 0 0 0 0 0.020641 0.032068 0.032068 0.032068 0.032068
  spline S145 degree 3 poles (-47.9282, -5.1269) (-47.9233, -5.3488) (-47.9147, -5.74) (-47.6813, -6.05) (-47.5803, -6.1842) knots 0 0 0 0 0.064538 0.113796 0.113796 0.113796 0.113796
  spline S146 degree 3 poles (-47.5803, -6.1842) (-47.3908, -6.3052) (-46.9667, -6.5759) (-46.4614, -6.5916) (-46.182, -6.6003) knots 0 0 0 0 0.066297 0.148303 0.148303 0.148303 0.148303
  spline S147 degree 3 poles (-46.182, -6.6003) (-45.9251, -6.5961) (-45.4728, -6.5887) (-45.0725, -6.3824) (-44.8995, -6.2933) knots 0 0 0 0 0.075765 0.133425 0.133425 0.133425 0.133425
  spline S148 degree 3 poles (-44.8995, -6.2933) (-44.769, -6.161) (-44.4723, -5.8602) (-44.357, -5.4514) (-44.2925, -5.2224) knots 0 0 0 0 0.054917 0.124877 0.124877 0.124877 0.124877
  line L103 (-44.2925, -5.2224) -> (-43.0919, -5.3861)
  spline S149 degree 3 poles (-43.0919, -5.3861) (-43.1504, -5.6241) (-43.2597, -6.0691) (-43.513, -6.4503) (-43.6308, -6.6276) knots 0 0 0 0 0.07287 0.136248 0.136248 0.136248 0.136248
  spline S150 degree 3 poles (-43.6308, -6.6276) (-43.7759, -6.7794) (-44.0835, -7.1015) (-44.4969, -7.2689) (-44.7154, -7.3575) knots 0 0 0 0 0.062278 0.132061 0.132061 0.132061 0.132061
  spline S151 degree 3 poles (-44.7154, -7.3575) (-44.9689, -7.433) (-45.5049, -7.5927) (-46.0644, -7.6084) (-46.3593, -7.6167) knots 0 0 0 0 0.078998 0.167061 0.167061 0.167061 0.167061
  spline S152 degree 3 poles (-46.3593, -7.6167) (-46.6416, -7.6119) (-47.154, -7.6033) (-47.6459, -7.4619) (-47.8668, -7.3984) knots 0 0 0 0 0.08425 0.152908 0.152908 0.152908 0.152908
  spline S153 degree 3 poles (-47.8668, -7.3984) (-48.0419, -7.327) (-48.3619, -7.1966) (-48.608, -6.9552) (-48.7195, -6.8459) knots 0 0 0 0 0.056055 0.102466 0.102466 0.102466 0.102466
  spline S154 degree 3 poles (-48.7195, -6.8459) (-48.8044, -6.7255) (-48.9832, -6.4721) (-49.0607, -6.1715) (-49.1015, -6.0137) knots 0 0 0 0 0.043817 0.092244 0.092244 0.092244 0.092244
  spline S155 degree 3 poles (-49.1015, -6.0137) (-49.1192, -5.8672) (-49.1646, -5.4913) (-49.1635, -5.1125) (-49.1629, -4.8813) knots 0 0 0 0 0.044238 0.113491 0.113491 0.113491 0.113491
  line L104 (-49.1629, -4.8813) -> (-49.1629, -3.2442)
  spline S156 degree 3 poles (-49.1629, -3.2442) (-49.1602, -2.7777) (-49.156, -2.0534) (-49.2164, -1.3319) (-49.2379, -1.075) knots 0 0 0 0 0.139849 0.217135 0.217135 0.217135 0.217135
  spline S157 degree 3 poles (-49.2379, -1.075) (-49.2718, -0.9257) (-49.3404, -0.6239) (-49.4808, -0.3481) (-49.5517, -0.2087) knots 0 0 0 0 0.045752 0.092454 0.092454 0.092454 0.092454
  line L105 (-49.5517, -0.2087) -> (-48.2693, -0.2087)
  spline S158 degree 3 poles (-48.2693, -0.2087) (-48.2109, -0.3452) (-48.0884, -0.6317) (-48.0459, -0.9406) (-48.0237, -1.1023) knots 0 0 0 0 0.04431 0.093043 0.093043 0.093043 0.093043
  circle A46 centre (-48.3914, 7.0872) radius 4.5
  dimension "d39" = 9
  constraint concentric A45 A46
  measures "d39" diameter of A46
delete_face "DeleteFace4" 1 faces at (43.665, -6.6143, 0.5)
extrude "Extrude11" cut sketch "Sketch14" against normal blind 14.5 contours A46
